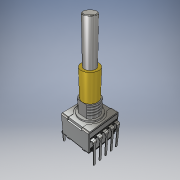
# Autodesk Inventor part: ELMA-E37
Saved by Autodesk Inventor 2018 (Build 220112000, 112)
## iProperties
Created: 2020-04-23
Part Number: ELMA-E37
Material: Všeobecné
Document SubType Name: Modeling
Designer: Jozko Mrkvicka
Density: 1 g/cm^3
Appearance: Výchozí
Author: Jozko Mrkvicka
Autodesk Inventor part; units mm, degrees
ref_plane "YZ Plane" through (0, 0, 0) normal (1, 0, 0) x (0, 1, 0)
ref_plane "XZ Plane" through (0, 0, 0) normal (0, 1, 0) x (-1, 0, 0)
sketch "Náčrt1" plane through (0, 0, 0) normal (0, 1, 0) x (-1, 0, 0)
  line L0 (-5.75, 6.25) -> (5.75, 6.25)
  line L1 (5.75, 6.25) -> (5.75, -6.25)
  line L2 (5.75, -6.25) -> (-5.75, -6.25)
  line L3 (-5.75, -6.25) -> (-5.75, 6.25)
  line L4 (-5.75, 6.25) -> (5.75, -6.25) construction
  line L5 (5.75, 6.25) -> (-5.75, -6.25) construction
  point P0 (0, 0)
  dimension "d0" = 11.5
  dimension "d1" = 12.5
  constraints: 12 end point, 2 midpoint, 2 parallel, 1 horizontal, 1 perpendicular
  measures "d0" distance of L1.end L2.end
  measures "d1" distance of L0.end L1.end
extrude "Vysunutí1" add sketch "Náčrt1" along normal blind 9
sketch "Náčrt2" plane through (0, 9, 0) normal (0, 1, 0) x (1, 0, 0)
  circle A0 centre (0, 0) radius 4.25
  dimension "d4" = 8.5
  constraints: 1 centre point, 1 coincident
  measures "d4" diameter of A0
extrude "Vysunutí2" add sketch "Náčrt2" along normal blind 0.5
sketch "Náčrt3" plane through (0, 9, 0) normal (0, 1, 0) x (1, 0, 0)
  circle A0 centre (0, 0) radius 4.25 projected
  line L0 (5.75, 6.25) -> (-5.75, 6.25) projected
  line L1 (3, -6.25) -> (-3, -6.25)
  line L2 (-3, 6.25) -> (3, 6.25)
  line L3 (-3, -6.25) -> (-3, -4)
  line L4 (-3, 4) -> (-3, 6.25)
  arc A1 (3, -4) -> (3, 4) centre (0, 0) ccw
  arc A2 (-3, 4) -> (-3, -4) centre (0, 0) ccw
  line L5 (3, 6.25) -> (3, 4)
  line L6 (3, -4) -> (3, -6.25)
  constraints: 12 end point, 5 parallel, 4 point on circle, 2 centre point, 2 perpendicular, 1 coincident, 1 horizontal, 1 point on line
extrude "Vysunutí3" cut sketch "Náčrt3" against normal blind 0.1
sketch "Náčrt4" plane through (0, 8.9, 0) normal (0, 1, 0) x (1, 0, 0)
  line L0 (3, 6.25) -> (3, 4) projected
  line L1 (3, -4) -> (3, -6.25) projected
  line L2 (-3, -6.25) -> (3, -6.25)
  line L3 (3, -6.25) -> (3, -5.75)
  line L4 (3, -5.75) -> (-3, -5.75)
  line L5 (-3, -5.75) -> (-3, -6.25)
  line L6 (-3, 6.25) -> (3, 6.25)
  line L7 (3, 6.25) -> (3, 5.75)
  line L8 (3, 5.75) -> (-3, 5.75)
  line L9 (-3, 5.75) -> (-3, 6.25)
  constraints: 16 end point, 4 parallel, 2 horizontal, 2 perpendicular, 2 point on line
extrude "Vysunutí4" cut sketch "Náčrt4" against normal blind 1
fillet "Zaoblení1" radius 0.5 4 edges at (4.375, 9, 6.25) (-4.375, 9, 6.25) (4.375, 9, -6.25) (-4.375, 9, -6.25)
sketch "Náčrt5" plane through (0, 9.5, 0) normal (0, 1, 0) x (1, 0, 0)
  circle A0 centre (0, 0) radius 4.25 projected
  circle A1 centre (0, 0) radius 3.5
  dimension "d16" = 7
  constraints: 1 centre point, 1 coincident
  measures "d16" diameter of A1
extrude "Vysunutí5" add sketch "Náčrt5" along normal blind 5 contours A1
sketch "Náčrt6" plane through (0, 14.5, 0) normal (0, 1, 0) x (1, 0, 0)
  circle A0 centre (0, 0) radius 3.5 projected
  line L0 (1.8028, 3) -> (-1.8028, 3)
  line L1 (-1.8028, -3) -> (1.8028, -3)
  arc A1 (1.8028, 3) -> (-1.8028, 3) centre (0, 0) ccw
  arc A2 (-1.8028, -3) -> (1.8028, -3) centre (0, 0) ccw
  constraints: 4 end point, 4 point on circle, 2 centre point, 1 coincident, 1 horizontal, 1 parallel
extrude "Vysunutí6" cut sketch "Náčrt6" against normal blind 5 contours L0 A0 | A0 L1
sketch "Náčrt7" plane through (0, 14.5, 0) normal (0, 1, 0) x (1, 0, 0)
  arc A0 (1.8028, -3) -> (1.8028, 3) centre (0, 0) ccw projected
  circle A1 centre (0, 0) radius 3
  dimension "d22" = 6
  constraints: 1 centre point, 1 coincident
  measures "d22" diameter of A1
extrude "Vysunutí7" add sketch "Náčrt7" along normal blind 10
sketch "Náčrt8" plane through (0, 24.5, 0) normal (0, 1, 0) x (1, 0, 0)
  circle A0 centre (0, 0) radius 3 projected
  circle A1 centre (0, 0) radius 2
  dimension "d25" = 4
  constraints: 1 centre point, 1 coincident
  measures "d25" diameter of A1
extrude "Vysunutí8" add sketch "Náčrt8" along normal blind 14 contours A1
chamfer "Zkosení1" distance 0.2 angle 45 1 edges at (-2, 38.5, 0)
thread "Závit3" size "M7x1" class "6g" standard "ANSI Metric M Profile" length 4
thread "Závit4" size "M7x1" class "6g" standard "ANSI Metric M Profile" length 4
sketch "Náčrt9" plane through (0, 0, 0) normal (0, -1, 0) x (1, 0, 0)
  line L0 (5.75, -6.25) -> (5.75, 6.25) projected
  line L1 (5.75, 6.25) -> (5.75, 5.75)
  line L2 (-5.75, 5.75) -> (-5.75, 6.25)
  line L3 (-3, 6.25) -> (-3, 5.75)
  line L4 (-4, 5.75) -> (-4, 6.25)
  line L5 (5.75, 5.75) -> (3, 5.75) projected
  line L6 (3, 6.25) -> (3, 5.75)
  line L7 (4, 5.75) -> (4, 6.25)
  line L8 (5.75, -5.75) -> (5.75, -6.25)
  line L9 (-5.75, -6.25) -> (-5.75, -5.75)
  line L10 (-3, -5.75) -> (-3, -6.25)
  line L11 (-4, -6.25) -> (-4, -5.75)
  line L12 (3, -5.75) -> (3, -6.25)
  line L13 (4, -6.25) -> (4, -5.75)
  line L14 (5.75, -6.25) -> (4, -6.25)
  line L15 (4, -5.75) -> (5.75, -5.75)
  line L16 (-5.75, -5.75) -> (-4, -5.75)
  line L17 (-3, -5.75) -> (3, -5.75)
  line L18 (3, -6.25) -> (-3, -6.25)
  line L19 (-4, -6.25) -> (-5.75, -6.25)
  line L20 (-4, 5.75) -> (-5.75, 5.75)
  line L21 (-5.75, 6.25) -> (-4, 6.25)
  line L22 (5.75, 5.75) -> (4, 5.75)
  line L23 (3, 5.75) -> (-3, 5.75)
  line L24 (-3, 6.25) -> (3, 6.25)
  line L25 (4, 6.25) -> (5.75, 6.25)
  point P0 (0, 0)
  constraints: 48 end point, 24 parallel, 6 horizontal, 6 perpendicular, 1 point on line
extrude "Vysunutí9" cut sketch "Náčrt9" against normal blind 1
sketch "Náčrt10" plane through (0, 0, 0) normal (0, -1, 0) x (1, 0, 0)
  line L0 (-3, 5.75) -> (-3, 6.25) projected
  line L1 (-4, 6.25) -> (-4, 5.75) projected
  line L2 (-4, 5.75) -> (-4.5, 5.375)
  line L3 (-4.5, 5) -> (-2.5, 5)
  line L4 (-3, 5.75) -> (-3, 6.25) projected
  line L5 (-2.5, 5.375) -> (-3, 5.75)
  line L6 (-2.5, 5.375) -> (-2.5, 5)
  line L7 (-2.5, 5) -> (-4.5, 5)
  line L8 (-4.5, 5) -> (-4.5, 5.375)
  line L9 (-4, 6.25) -> (-4, 5.75) projected
  line L10 (-4, 5.75) -> (-4, 6.25)
  line L11 (-4, 6.25) -> (-3, 6.25)
  line L12 (-3, 6.25) -> (-3, 5.75)
  line L13 (3, 5.75) -> (2.5, 5.375)
  line L14 (2.5, 5) -> (4.5, 5)
  line L15 (4.5, 5.375) -> (4, 5.75)
  line L16 (4.5, 5.375) -> (4.5, 5)
  line L17 (4.5, 5) -> (2.5, 5)
  line L18 (2.5, 5) -> (2.5, 5.375)
  line L19 (3, 5.75) -> (3, 6.25)
  line L20 (3, 6.25) -> (4, 6.25)
  line L21 (4, 6.25) -> (4, 5.75)
  line L22 (3, -6.25) -> (3, -5.75)
  line L23 (2.5, -5.375) -> (3, -5.75)
  line L24 (4, -5.75) -> (4, -6.25)
  line L25 (4, -6.25) -> (3, -6.25)
  line L26 (4, -5.75) -> (4.5, -5.375)
  line L27 (4.5, -5) -> (2.5, -5)
  line L28 (2.5, -5) -> (4.5, -5)
  line L29 (4.5, -5) -> (4.5, -5.375)
  line L30 (2.5, -5.375) -> (2.5, -5)
  line L31 (-4, -6.25) -> (-4, -5.75)
  line L32 (-4.5, -5.375) -> (-4, -5.75)
  line L33 (-3, -5.75) -> (-3, -6.25)
  line L34 (-3, -6.25) -> (-4, -6.25)
  line L35 (-3, -5.75) -> (-2.5, -5.375)
  line L36 (-2.5, -5) -> (-2.5, -5.375)
  line L37 (-4.5, -5.375) -> (-4.5, -5)
  line L38 (-4.5, 5) -> (-2.5, 5)
  line L39 (2.5, 5) -> (4.5, 5)
  line L40 (2.5, -5) -> (4.5, -5)
  line L41 (-4.5, -5) -> (-2.5, -5)
  point P0 (0, 0)
  constraints: 76 end point, 8 perpendicular, 5 equal length, 4 horizontal
extrude "Vysunutí11" add sketch "Náčrt10" along normal blind 0.2
fillet "Zaoblení2" radius 0.8 4 edges at (-3.5, -0.2, 6.25) (3.5, -0.2, 6.25) (-3.5, -0.2, -6.25) (3.5, -0.2, -6.25)
sketch "Náčrt11" plane through (-5.75, 9, -5.75) normal (-1, 0, 0) x (0, 0, 1)
  line L0 (-0.5, -8) -> (0, -8) projected
  line L1 (12, -8) -> (12, 0)
  line L2 (12, 0) -> (-0.5, 0)
  line L3 (-0.5, 0) -> (-0.5, -8)
  line L4 (0, -0.5) -> (11.5, -0.5)
  line L5 (11.5, -0.5) -> (11.5, -8)
  line L6 (0, -8) -> (0, -0.5)
  line L7 (-0.5, -8) -> (0, -8)
  line L8 (11.5, -8) -> (12, -8)
  point P0 (12, -8)
  point P1 (12, -0.5)
  point P2 (-0.5, -0.5)
  constraints: 16 end point, 4 parallel, 3 horizontal, 3 perpendicular
extrude "Vysunutí12" cut sketch "Náčrt11" against normal blind 0.1
sketch "Náčrt12" plane through (5.75, 9, 5.75) normal (1, 0, 0) x (0, 0, -1)
  arc A0 (0, 0) -> (-0.5, -0.5) centre (0, -0.5) ccw projected
  line L0 (11.5, 0) -> (0, 0) projected
  arc A1 (12, -0.5) -> (11.5, 0) centre (11.5, -0.5) ccw projected
  line L1 (12, -8) -> (12, -0.5) projected
  line L2 (11.5, -8) -> (12, -8) projected
  line L3 (11.5, -0.5) -> (11.5, -8) projected
  line L4 (0, -0.5) -> (11.5, -0.5) projected
  line L5 (0, -8) -> (0, -0.5) projected
  line L6 (-0.5, -8) -> (0, -8) projected
  line L7 (-0.5, -0.5) -> (-0.5, -8) projected
  point P0 (5.75, -9)
extrude "Vysunutí13" cut sketch "Náčrt12" against normal blind 0.1
sketch "Náčrt13" plane through (-5.75, 0, -5.75) normal (-1, 0, 0) x (0, 0, 1)
  line L0 (11.5, 0) -> (11.5, 8.5) projected
  line L1 (0, 8.5) -> (11.5, 8.5)
  line L2 (11.5, 8.5) -> (11.5, 6)
  line L3 (0, 6) -> (0, 8.5)
  line L4 (11.5, 6) -> (11.5, 3.5)
  line L5 (11.5, 3.5) -> (0, 3.5)
  line L6 (0, 3.5) -> (0, 6)
  line L7 (0, 3.5) -> (11.5, 3.5)
  line L8 (11.5, 3.5) -> (11.5, 4)
  line L9 (9.75, 4) -> (1.75, 4)
  line L10 (0, 4) -> (0, 3.5)
  line L11 (9.75, 4) -> (1.75, 4)
  line L12 (9.75, 4) -> (10.1027, 6)
  line L13 (1.75, 4) -> (1.3973, 6)
  line L14 (1.75, 4) -> (3.7809, 4) construction
  line L15 (11.5, 6) -> (10.1027, 6)
  line L16 (1.3973, 6) -> (0, 6)
  line L17 (0, 6) -> (1.3973, 6)
  line L18 (10.1027, 6) -> (11.5, 6)
  point P0 (5.75, 0)
  point P1 (5.75, 5)
  constraints: 36 end point, 8 parallel, 5 horizontal, 4 perpendicular, 3 point on line, 1 equal length
extrude "Vysunutí14" cut sketch "Náčrt13" against normal blind 0.5 contours L5 L6 L16 L13 L9 L12 L15 L0
sketch "Náčrt14" plane through (-5.25, 0, -5.75) normal (-1, 0, 0) x (0, 0, 1)
  line L0 (9.75, 4) -> (10.1027, 6) projected
  line L1 (1.3973, 6) -> (1.75, 4) projected
  line L2 (0, 6) -> (1.3973, 6) projected
  line L3 (0, 3.5) -> (0, 6) projected
  line L4 (11.5, 6) -> (11.5, 3.5) projected
  line L5 (10.1027, 6) -> (11.5, 6) projected
  line L6 (0, 6) -> (11.5, 6)
  line L7 (11.5, 6) -> (11.5, 3.5)
  line L8 (11.5, 3.5) -> (0, 3.5)
  line L9 (0, 3.5) -> (0, 6)
  line L10 (9.75, 4) -> (1.75, 4)
  line L11 (0.5, 5.5) -> (0, 5.5)
  line L12 (1.25, 4) -> (0.9855, 5.5)
  line L13 (1.25, 4) -> (1.3382, 3.5)
  line L14 (10.25, 4) -> (10.5145, 5.5)
  line L15 (10.25, 4) -> (10.1618, 3.5)
  line L16 (11, 5.5) -> (11.5, 5.5)
  line L17 (0.5, 5.5) -> (0.9855, 5.5)
  line L18 (10.5145, 5.5) -> (11, 5.5)
  point P0 (5.75, 0)
  point P1 (0.5, 4)
  constraints: 26 end point, 6 point on line, 5 parallel, 3 horizontal, 3 perpendicular
extrude "Vysunutí15" add sketch "Náčrt14" along normal blind 0.45 contours L0 L5 L4 L16 L18 L14 L15 L8 L13 L12 L17 L11 L3 L2 L1 L10
sketch "Náčrt15" plane through (-5.75, 0, -5.75) normal (-1, 0, 0) x (0, 0, 1)
  line L0 (11.5, 1) -> (11.5, 3.5) projected
  line L1 (0, 0) -> (11.5, 0)
  line L2 (11.5, 0) -> (11.5, 1.5)
  line L3 (11.5, 1.5) -> (0, 1.5)
  line L4 (0, 1.5) -> (0, 0)
  line L5 (11.5, 3.5) -> (0, 3.5) projected
  point P0 (5.75, 0)
  constraints: 8 end point, 2 parallel, 1 horizontal, 1 perpendicular, 1 point on line
extrude "Vysunutí16" cut sketch "Náčrt15" against normal blind 0.05
chamfer "Zkosení2" distance 0.05 angle 45 1 edges at (-5.7, 5.75, -5.75)
chamfer "Zkosení3" distance 0.05 angle 45 1 edges at (-5.7, 5.75, 5.75)
chamfer "Zkosení4" distance 0.05 angle 45 1 edges at (-5.7, 0.75, -5.75)
chamfer "Zkosení5" distance 0.05 angle 45 1 edges at (-5.7, 0.75, 5.75)
sketch "Náčrt17" plane through (5.75, 0, 5.75) normal (1, 0, 0) x (0, 0, -1)
  line L0 (11.5, 0) -> (11.5, 8.5) projected
  line L1 (0, 8.5) -> (11.5, 8.5)
  line L2 (11.5, 8.5) -> (11.5, 6.5)
  line L3 (11.5, 6.5) -> (0, 6.5)
  line L4 (0, 6.5) -> (0, 8.5)
  line L5 (0, 6.5) -> (11.5, 6.5)
  line L6 (11.5, 6.5) -> (11.5, 5)
  line L7 (11.5, 5) -> (0, 5)
  line L8 (0, 5) -> (0, 6.5)
  point P0 (5.75, 0)
  constraints: 16 end point, 4 parallel, 2 horizontal, 2 perpendicular, 2 point on line
extrude "Vysunutí18" cut sketch "Náčrt17" against normal blind 0.05 contours L7 L8 L3 L0
sketch "Náčrt18" plane through (5.75, 0, 5.75) normal (1, 0, 0) x (0, 0, -1)
  line L0 (0, 8.5) -> (0, 1) projected
  line L1 (11.5, 0) -> (11.5, 5) projected
  line L2 (1.3973, 2.5) -> (1.75, 0.5)
  line L3 (10.1027, 2.5) -> (9.75, 0.5)
  line L4 (1.75, 0.5) -> (9.75, 0.5)
  line L5 (11.5, 2.5) -> (11.5, 0)
  line L6 (11.5, 0) -> (0, 0)
  line L7 (0, 0) -> (0, 2.5)
  line L8 (0, 2.5) -> (1.3973, 2.5)
  line L9 (10.1027, 2.5) -> (11.5, 2.5)
  line L10 (11.5, 2.5) -> (11.5, 0)
  constraints: 20 end point, 3 horizontal, 3 parallel, 2 perpendicular, 1 collinear, 1 point on line
extrude "Vysunutí19" cut sketch "Náčrt18" against normal blind 0.5
chamfer "Zkosení8" distance 0.05 angle 45 1 edges at (5.7, 5.75, 5.75)
chamfer "Zkosení9" distance 0.05 angle 45 1 edges at (5.7, 5.75, -5.75)
sketch "Náčrt19" plane through (5.25, 0, 5.75) normal (1, 0, 0) x (0, 0, -1)
  line L0 (11.5, 2.5) -> (11.5, 1) projected
  line L1 (10.1027, 2.5) -> (11.5, 2.5) projected
  line L2 (9.75, 0.5) -> (10.1027, 2.5) projected
  line L3 (1.75, 0.5) -> (9.75, 0.5) projected
  line L4 (1.3973, 2.5) -> (1.75, 0.5) projected
  line L5 (0, 2.5) -> (1.3973, 2.5) projected
  line L6 (11.5, 0) -> (0, 0) projected
  line L7 (0, 2.5) -> (11.5, 2.5)
  line L8 (11.5, 2.5) -> (11.5, 2)
  line L9 (0, 2) -> (0, 2.5)
  line L10 (1.25, 0.5) -> (1, 2)
  line L11 (1.25, 0.5) -> (1.3333, 0)
  line L12 (10.2497, 0.5) -> (10.5142, 2)
  line L13 (10.2497, 0.5) -> (10.1616, 0)
  line L14 (11.5, 2) -> (10.5142, 2)
  line L15 (1, 2) -> (0, 2)
  point P0 (5.75, 0)
  constraints: 18 end point, 5 point on line, 4 parallel, 1 horizontal, 1 perpendicular
extrude "Vysunutí20" add sketch "Náčrt19" along normal blind 0.45 contours L0 L14 L12 L13 L6 L11 L10 L15 L9 L5 L4 L3 L2 L1
chamfer "Zkosení10" distance 0.05 angle 45 1 edges at (5.7, 2.25, 5.75)
chamfer "Zkosení11" distance 0.05 angle 45 1 edges at (5.7, 2.25, -5.75)
sketch "Náčrt20" plane through (-5.7, 0, -5.75) normal (-1, 0, 0) x (0, 0, 1)
  line L0 (11.45, 1.5) -> (11.45, 0) projected
  line L1 (0.05, 1.5) -> (11.45, 1.5) projected
  line L2 (0.05, 0) -> (0.05, 1.5) projected
  line L3 (5.75, 0.75) -> (8.29, 0.75)
  line L4 (5.75, 0.75) -> (8.29, 0.75) construction
  line L5 (8.29, 0.75) -> (10.83, 0.75)
  line L6 (5.75, 0.75) -> (3.21, 0.75)
  line L7 (3.21, 0.75) -> (0.67, 0.75)
  line L8 (6.5, 0.65) -> (5, 0.65)
  line L9 (5, 0.65) -> (5, 0.85)
  line L10 (5, 0.85) -> (6.5, 0.85)
  line L11 (6.5, 0.85) -> (6.5, 0.65)
  line L12 (6.5, 0.65) -> (5, 0.85) construction
  line L13 (5, 0.65) -> (6.5, 0.85) construction
  line L14 (9.04, 0.65) -> (7.54, 0.65)
  line L15 (7.54, 0.65) -> (7.54, 0.85)
  line L16 (7.54, 0.85) -> (9.04, 0.85)
  line L17 (9.04, 0.85) -> (9.04, 0.65)
  line L18 (9.04, 0.65) -> (7.54, 0.85) construction
  line L19 (7.54, 0.65) -> (9.04, 0.85) construction
  line L20 (11.45, 0.65) -> (10.08, 0.65)
  line L21 (10.08, 0.65) -> (10.08, 0.85)
  line L22 (10.08, 0.85) -> (11.45, 0.85)
  line L23 (3.96, 0.65) -> (2.46, 0.65)
  line L24 (2.46, 0.65) -> (2.46, 0.85)
  line L25 (2.46, 0.85) -> (3.96, 0.85)
  line L26 (3.96, 0.85) -> (3.96, 0.65)
  line L27 (3.96, 0.65) -> (2.46, 0.85) construction
  line L28 (2.46, 0.65) -> (3.96, 0.85) construction
  line L29 (1.42, 0.65) -> (0.05, 0.65)
  line L30 (0.05, 0.85) -> (1.42, 0.85)
  line L31 (1.42, 0.85) -> (1.42, 0.65)
  line L32 (0.05, 0.85) -> (0.05, 0.65)
  line L33 (11.45, 0.85) -> (11.45, 0.65)
  point P0 (5.75, 0)
  point P1 (5.75, 1.5)
  point P2 (10.83, 0.75)
  point P3 (3.21, 0.75)
  point P4 (0.67, 0.75)
  constraints: 62 end point, 8 horizontal, 8 parallel, 7 midpoint, 6 point on line, 4 perpendicular, 1 collinear
extrude "Vysunutí21" add sketch "Náčrt20" along normal blind 1.25 contours L0 L20 L21 L22 | L30 L31 L29 L2 | L17 L14 L15 L3 L5 | L5 L3 L15 L16 L17 | L24 L25 L26 L6 L7 | L7 L6 L26 L23 L24 | L11 L8 L9 L6 L3 | L3 L6 L9 L10 L11
sketch "Náčrt21" plane through (-5.7, 0.65, -0.75) normal (0, -1, 0) x (1, 0, 0)
  line L0 (0, 1.5) -> (-1.25, 1.5) projected
  line L1 (-1.25, 0) -> (-1.25, 1.5) projected
  line L2 (-1.25, 0) -> (-1.05, 0)
  line L3 (-1.05, 0) -> (-1.05, 1.5)
  line L4 (-1.05, 1.5) -> (-1.25, 1.5)
  line L5 (-1.25, 1.5) -> (-1.25, 0)
  line L6 (0, -2.54) -> (-1.25, -2.54) projected
  line L7 (0, 2.54) -> (-1.25, 2.54) projected
  line L8 (-1.25, -2.54) -> (-1.05, -2.54)
  line L9 (-1.05, -2.54) -> (-1.05, -1.04)
  line L10 (-1.05, -1.04) -> (-1.25, -1.04)
  line L11 (-1.25, -1.04) -> (-1.25, -2.54)
  line L12 (-1.25, 2.54) -> (-1.05, 2.54)
  line L13 (-1.05, 2.54) -> (-1.05, 4.04)
  line L14 (-1.05, 4.04) -> (-1.25, 4.04)
  line L15 (-1.25, 4.04) -> (-1.25, 2.54)
  line L16 (-1.25, -4.95) -> (-1.25, -3.58) projected
  line L17 (0, -4.95) -> (-1.25, -4.95) projected
  line L18 (-1.25, -3.58) -> (-1.05, -3.58)
  line L19 (-1.05, -3.58) -> (-1.05, -4.95)
  line L20 (-1.05, -4.95) -> (-1.25, -4.95)
  line L21 (-1.25, -4.95) -> (-1.25, -3.58)
  line L22 (0, 5.08) -> (-1.25, 5.08) projected
  line L23 (0, 6.45) -> (-1.25, 6.45) projected
  line L24 (-1.25, 5.08) -> (-1.05, 5.08)
  line L25 (-1.05, 5.08) -> (-1.05, 6.45)
  line L26 (-1.05, 6.45) -> (-1.25, 6.45)
  line L27 (-1.25, 6.45) -> (-1.25, 5.08)
  point P0 (5.7, 0.75)
  constraints: 40 end point, 10 parallel, 5 horizontal, 5 perpendicular, 4 point on line
extrude "Vysunutí22" add sketch "Náčrt21" along normal blind 1
sketch "Náčrt22" plane through (-5.7, -0.35, -0.75) normal (0, -1, 0) x (1, 0, 0)
  line L0 (-1.25, 0.35) -> (-1.05, 0.35)
  line L1 (-1.05, 0.35) -> (-1.05, 1.15)
  line L2 (-1.05, 1.15) -> (-1.25, 1.15)
  line L3 (-1.25, 1.15) -> (-1.25, 0.35)
  line L4 (-1.25, -2.19) -> (-1.05, -2.19)
  line L5 (-1.05, -2.19) -> (-1.05, -1.39)
  line L6 (-1.05, -1.39) -> (-1.25, -1.39)
  line L7 (-1.25, -1.39) -> (-1.25, -2.19)
  line L8 (-1.25, 2.89) -> (-1.05, 2.89)
  line L9 (-1.05, 2.89) -> (-1.05, 3.69)
  line L10 (-1.05, 3.69) -> (-1.25, 3.69)
  line L11 (-1.25, 3.69) -> (-1.25, 2.89)
  line L12 (-1.25, 5.43) -> (-1.05, 5.43)
  line L13 (-1.05, 5.43) -> (-1.05, 6.23)
  line L14 (-1.05, 6.23) -> (-1.25, 6.23)
  line L15 (-1.25, 6.23) -> (-1.25, 5.43)
  line L16 (-1.25, -4.73) -> (-1.05, -4.73)
  line L17 (-1.05, -4.73) -> (-1.05, -3.93)
  line L18 (-1.05, -3.93) -> (-1.25, -3.93)
  line L19 (-1.25, -3.93) -> (-1.25, -4.73)
  point P0 (5.7, 0.75)
  point P1 (-1.15, 0.75)
  point P2 (-1.15, -1.79)
  point P3 (-1.15, 3.29)
  point P4 (-1.15, 5.83)
  point P5 (-1.15, -4.33)
  point P6 (-1.15, -1.79)
  point P7 (-1.15, 3.29)
  point P8 (-1.15, 5.83)
  point P9 (-1.15, -4.33)
  constraints: 40 end point, 10 parallel, 5 horizontal, 5 perpendicular
extrude "Vysunutí23" add sketch "Náčrt22" along normal blind 4
chamfer "Zkosení12" distance 0.35 angle 45 1 edges at (-6.85, -0.35, -0.75) measured on face at (-6.85, -0.35, -0.65)
chamfer "Zkosení13" distance 0.35 angle 45 1 edges at (-6.85, -0.35, 0.75) measured on face at (-6.85, -0.35, 0.65)
chamfer "Zkosení14" distance 0.35 angle 45 1 edges at (-6.85, -0.35, 1.79) measured on face at (-6.85, -0.35, 1.89)
chamfer "Zkosení15" distance 0.35 angle 45 1 edges at (-6.85, -0.35, 3.29) measured on face at (-6.85, -0.35, 3.19)
chamfer "Zkosení16" distance 0.35 angle 45 1 edges at (-6.85, -0.35, 4.33) measured on face at (-6.85, -0.35, 4.43)
chamfer "Zkosení17" distance 0.22 angle 45 1 edges at (-6.85, -0.35, 5.7) measured on face at (-6.85, -0.35, 5.6)
chamfer "Zkosení18" distance 0.22 angle 45 1 edges at (-6.85, -0.35, -5.7) measured on face at (-6.85, -0.35, -5.6)
chamfer "Zkosení19" distance 0.35 angle 45 1 edges at (-6.85, -0.35, -4.33) measured on face at (-6.85, -0.35, -4.43)
chamfer "Zkosení20" distance 0.35 angle 45 1 edges at (-6.85, -0.35, -3.29) measured on face at (-6.85, -0.35, -3.19)
chamfer "Zkosení21" distance 0.35 angle 45 1 edges at (-6.85, -0.35, -1.79) measured on face at (-6.85, -0.35, -1.89)
fillet "Zaoblení3" radius 0.4 10 edges at (-6.85, -4.35, -5.48) (-6.85, -4.35, -4.68) (-6.85, -4.35, -2.94) (-6.85, -4.35, -2.14) (-6.85, -4.35, -0.4) (-6.85, -4.35, 0.4) (-6.85, -4.35, 2.14) (-6.85, -4.35, 2.94) (-6.85, -4.35, 4.68) (-6.85, -4.35, 5.48)
sketch "Náčrt23" plane through (5.7, 0, 5.75) normal (1, 0, 0) x (0, 0, -1)
  line L0 (11.45, 6.5) -> (11.45, 5) projected
  line L1 (0.05, 6.5) -> (11.45, 6.5) projected
  line L2 (0.05, 5) -> (0.05, 6.5) projected
  line L3 (11.45, 5) -> (0.05, 5) projected
  line L4 (11.45, 0.85) -> (10.08, 0.85) projected
  line L5 (10.08, 0.85) -> (10.08, 0.65) projected
  line L6 (9.04, 0.65) -> (9.04, 0.85) projected
  line L7 (9.04, 0.85) -> (7.54, 0.85) projected
  line L8 (7.54, 0.85) -> (7.54, 0.65) projected
  line L9 (7.54, 0.65) -> (9.04, 0.65) projected
  line L10 (6.5, 0.65) -> (6.5, 0.85) projected
  line L11 (6.5, 0.85) -> (5, 0.85) projected
  line L12 (5, 0.85) -> (5, 0.65) projected
  line L13 (5, 0.65) -> (6.5, 0.65) projected
  line L14 (3.96, 0.65) -> (3.96, 0.85) projected
  line L15 (3.96, 0.85) -> (2.46, 0.85) projected
  line L16 (2.46, 0.85) -> (2.46, 0.65) projected
  line L17 (2.46, 0.65) -> (3.96, 0.65) projected
  line L18 (11.45, 0.85) -> (10.08, 0.85) projected
  line L19 (10.08, 0.85) -> (10.08, 0.65) projected
  line L20 (10.08, 0.65) -> (11.45, 0.65) projected
  line L21 (11.45, 0) -> (11.45, 0.65) projected
  line L22 (0.05, 0) -> (11.45, 0) projected
  line L23 (0.05, 0.65) -> (0.05, 0) projected
  line L24 (0.05, 0.65) -> (1.42, 0.65) projected
  line L25 (1.42, 0.65) -> (1.42, 0.85) projected
  line L26 (1.42, 0.85) -> (0.05, 0.85) projected
  line L27 (0.05, 1.5) -> (0.05, 0.85) projected
  line L28 (11.45, 1.5) -> (0.05, 1.5) projected
  line L29 (11.45, 0.85) -> (11.45, 1.5) projected
  line L30 (11.45, 5.85) -> (10.08, 5.85)
  line L31 (10.08, 5.85) -> (10.08, 5.65)
  line L32 (9.04, 5.65) -> (9.04, 5.85)
  line L33 (9.04, 5.85) -> (7.54, 5.85)
  line L34 (7.54, 5.85) -> (7.54, 5.65)
  line L35 (7.54, 5.65) -> (9.04, 5.65)
  line L36 (6.5, 5.65) -> (6.5, 5.85)
  line L37 (6.5, 5.85) -> (5, 5.85)
  line L38 (5, 5.85) -> (5, 5.65)
  line L39 (5, 5.65) -> (6.5, 5.65)
  line L40 (3.96, 5.65) -> (3.96, 5.85)
  line L41 (3.96, 5.85) -> (2.46, 5.85)
  line L42 (2.46, 5.85) -> (2.46, 5.65)
  line L43 (2.46, 5.65) -> (3.96, 5.65)
  line L44 (11.45, 5.85) -> (10.08, 5.85)
  line L45 (10.08, 5.85) -> (10.08, 5.65)
  line L46 (10.08, 5.65) -> (11.45, 5.65)
  line L47 (11.45, 5) -> (11.45, 5.65)
  line L48 (0.05, 5) -> (11.45, 5)
  line L49 (0.05, 5.65) -> (0.05, 5)
  line L50 (0.05, 5.65) -> (1.42, 5.65)
  line L51 (1.42, 5.65) -> (1.42, 5.85)
  line L52 (1.42, 5.85) -> (0.05, 5.85)
  line L53 (0.05, 6.5) -> (0.05, 5.85)
  line L54 (11.45, 6.5) -> (0.05, 6.5)
  line L55 (11.45, 5.85) -> (11.45, 6.5)
  point P0 (5.75, 0)
  point P1 (5.75, 5)
  constraints: 52 end point, 1 coincident
extrude "Vysunutí24" add sketch "Náčrt23" along normal blind 1.25 contours L0 L46 L31 L30 | L52 L51 L50 L2 | L35 L34 L33 L32 | L39 L38 L37 L36 | L43 L42 L41 L40
sketch "Náčrt24" plane through (5.7, 5.65, -0.75) normal (0, -1, 0) x (1, 0, 0)
  line L0 (0, 0) -> (1.25, 0) projected
  line L1 (1.25, 1.5) -> (1.25, 0) projected
  line L2 (0, 1.5) -> (1.25, 1.5) projected
  line L3 (1.25, 1.5) -> (1.05, 1.5)
  line L4 (1.05, 1.5) -> (1.05, 0)
  line L5 (1.05, 0) -> (1.25, 0)
  line L6 (1.25, 0) -> (1.25, 1.5)
  line L7 (1.25, -1.04) -> (1.25, -2.54) projected
  line L8 (1.25, -4.95) -> (1.25, -3.58) projected
  line L9 (1.25, 2.54) -> (1.25, 4.04) projected
  line L10 (0, 5.08) -> (1.25, 5.08) projected
  line L11 (1.25, -1.04) -> (1.05, -1.04)
  line L12 (1.05, -1.04) -> (1.05, -2.54)
  line L13 (1.05, -2.54) -> (1.25, -2.54)
  line L14 (1.25, -2.54) -> (1.25, -1.04)
  line L15 (1.25, 4.04) -> (1.05, 4.04)
  line L16 (1.05, 4.04) -> (1.05, 2.54)
  line L17 (1.05, 2.54) -> (1.25, 2.54)
  line L18 (1.25, 2.54) -> (1.25, 4.04)
  line L19 (1.25, 6.45) -> (0, 6.45) projected
  line L20 (1.25, 5.08) -> (1.05, 5.08)
  line L21 (1.05, 5.08) -> (1.05, 6.45)
  line L22 (1.05, 6.45) -> (1.25, 6.45)
  line L23 (1.25, 6.45) -> (1.25, 5.08)
  line L24 (1.25, -3.58) -> (1.25, -4.95) projected
  line L25 (0, -4.95) -> (1.25, -4.95) projected
  line L26 (1.25, -3.58) -> (1.05, -3.58)
  line L27 (1.05, -3.58) -> (1.05, -4.95)
  line L28 (1.05, -4.95) -> (1.25, -4.95)
  line L29 (1.25, -4.95) -> (1.25, -3.58)
  point P0 (-5.7, 0.75)
  constraints: 40 end point, 10 parallel, 5 horizontal, 5 perpendicular, 4 point on line
extrude "Vysunutí25" add sketch "Náčrt24" along normal blind 1
sketch "Náčrt25" plane through (5.7, 4.65, -0.75) normal (0, -1, 0) x (1, 0, 0)
  line L0 (1.05, 0.35) -> (1.25, 0.35)
  line L1 (1.25, 0.35) -> (1.25, 1.15)
  line L2 (1.25, 1.15) -> (1.05, 1.15)
  line L3 (1.05, 1.15) -> (1.05, 0.35)
  line L4 (1.05, -2.19) -> (1.25, -2.19)
  line L5 (1.25, -2.19) -> (1.25, -1.39)
  line L6 (1.25, -1.39) -> (1.05, -1.39)
  line L7 (1.05, -1.39) -> (1.05, -2.19)
  line L8 (1.05, 2.89) -> (1.25, 2.89)
  line L9 (1.25, 2.89) -> (1.25, 3.69)
  line L10 (1.25, 3.69) -> (1.05, 3.69)
  line L11 (1.05, 3.69) -> (1.05, 2.89)
  line L12 (1.05, 5.43) -> (1.25, 5.43)
  line L13 (1.25, 5.43) -> (1.25, 6.23)
  line L14 (1.25, 6.23) -> (1.05, 6.23)
  line L15 (1.05, 6.23) -> (1.05, 5.43)
  line L16 (1.05, -4.73) -> (1.25, -4.73)
  line L17 (1.25, -4.73) -> (1.25, -3.93)
  line L18 (1.25, -3.93) -> (1.05, -3.93)
  line L19 (1.05, -3.93) -> (1.05, -4.73)
  line L20 (-12.45, -4.73) -> (-12.65, -4.73) projected
  line L21 (-12.65, -3.93) -> (-12.45, -3.93) projected
  line L22 (-12.65, -1.39) -> (-12.45, -1.39) projected
  line L23 (-12.45, -2.19) -> (-12.65, -2.19) projected
  line L24 (-12.45, 0.35) -> (-12.65, 0.35) projected
  line L25 (-12.65, 1.15) -> (-12.45, 1.15) projected
  line L26 (-12.65, 3.69) -> (-12.45, 3.69) projected
  line L27 (-12.45, 2.89) -> (-12.65, 2.89) projected
  line L28 (-12.45, 5.43) -> (-12.65, 5.43) projected
  line L29 (-12.65, 6.23) -> (-12.45, 6.23) projected
  line L30 (-11.45, 6.5) -> (-11.45, -5) projected
  point P0 (-5.7, 0.75)
  point P1 (1.15, 0.75)
  point P2 (1.15, -1.79)
  point P3 (1.15, 3.29)
  point P4 (1.15, 5.83)
  point P5 (1.15, -4.33)
  point P6 (1.15, -1.79)
  point P7 (1.15, 3.29)
  point P8 (1.15, 5.83)
  point P9 (1.15, -4.33)
  point P10 (1.15, 0.75)
  point P11 (1.15, 0.75)
  constraints: 40 end point, 10 parallel, 5 horizontal, 5 perpendicular
ref_plane "Pracovní rovina1" through (-6.95, -4.35, -2.54) normal (0, -1, 0) x (1, 0, 0)
extrude "Vysunutí26" add sketch "Náčrt25" along normal up to surface (9 mm away)
fillet "Zaoblení5" radius 0.4 10 edges at (6.85, -4.35, 5.48) (6.85, -4.35, 4.68) (6.85, -4.35, 2.94) (6.85, -4.35, 2.14) (6.85, -4.35, 0.4) (6.85, -4.35, -0.4) (6.85, -4.35, -2.14) (6.85, -4.35, -2.94) (6.85, -4.35, -4.68) (6.85, -4.35, -5.48)
chamfer "Zkosení30" distance 0.35 angle 45 1 edges at (6.85, 4.65, 3.29) measured on face at (6.85, 4.65, 3.19)
chamfer "Zkosení31" distance 0.35 angle 45 1 edges at (6.85, 4.65, 1.79) measured on face at (6.85, 4.65, 1.89)
chamfer "Zkosení32" distance 0.35 angle 45 1 edges at (6.85, 4.65, 0.75) measured on face at (6.85, 4.65, 0.65)
chamfer "Zkosení33" distance 0.35 angle 45 1 edges at (6.85, 4.65, -0.75) measured on face at (6.85, 4.65, -0.65)
chamfer "Zkosení34" distance 0.35 angle 45 1 edges at (6.85, 4.65, 4.33) measured on face at (6.85, 4.65, 4.43)
chamfer "Zkosení35" distance 0.35 angle 45 1 edges at (6.85, 4.65, -1.79) measured on face at (6.85, 4.65, -1.89)
chamfer "Zkosení36" distance 0.35 angle 45 1 edges at (6.85, 4.65, -3.29) measured on face at (6.85, 4.65, -3.19)
chamfer "Zkosení37" distance 0.35 angle 45 1 edges at (6.85, 4.65, -4.33) measured on face at (6.85, 4.65, -4.43)
chamfer "Zkosení38" distance 0.22 angle 45 1 edges at (6.85, 4.65, -5.7) measured on face at (6.85, 4.65, -5.6)
chamfer "Zkosení39" distance 0.22 angle 45 1 edges at (6.85, 4.65, 5.7) measured on face at (6.85, 4.65, 5.6)
fillet "Zaoblení7" radius 0.5 10 edges at (6.95, 5.85, 5.015) (6.95, 5.85, 2.54) (6.95, 5.85, 0) (6.95, 5.85, -2.54) (6.95, 5.85, -5.015) (-6.95, 0.85, 5.015) (-6.95, 0.85, 2.54) (-6.95, 0.85, 0) (-6.95, 0.85, -2.54) (-6.95, 0.85, -5.015)
fillet "Zaoblení8" radius 0.3 1 edges at (6.75, 5.65, 5.015)
fillet "Zaoblení9" radius 0.3 9 edges at (-6.75, 0.65, 5.015) (-6.75, 0.65, 2.54) (-6.75, 0.65, 0) (-6.75, 0.65, -2.54) (-6.75, 0.65, -5.015) (6.75, 5.65, 2.54) (6.75, 5.65, 0) (6.75, 5.65, -2.54) (6.75, 5.65, -5.015)
